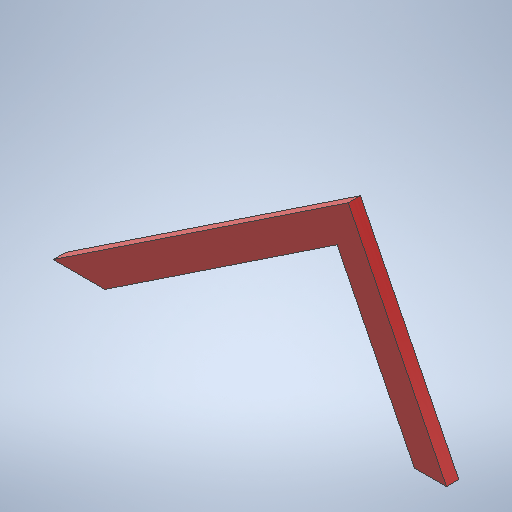
# Autodesk Inventor part: side1
Saved by Autodesk Inventor 2025.1 (Build 291241020, 241B)
## iProperties
Created: 2024-09-20
Part Number: side1
Material: Generic
Document SubType Name: Modeling
Designer: User
Density: 1 g/cm^3
Appearance: Default
Author: User
Autodesk Inventor part; units mm, degrees
ref_plane "YZ Plane" through (0, 0, 0) normal (1, 0, 0) x (0, 1, 0)
ref_plane "XZ Plane" through (0, 0, 0) normal (0, 1, 0) x (-1, 0, 0)
ref_plane "XY Plane" through (0, 0, 0) normal (0, 0, 1) x (1, 0, 0)
sketch "Sketch1" plane through (0, 0, 0) normal (0, 0, 1) x (1, 0, 0)
  line L0 (0, 0) -> (0, -38.1) projected
  line L1 (0, -38.1) -> (1219.2, -38.1) projected
  line L2 (1219.2, 0) -> (1219.2, -38.1) projected
  line L3 (0, 0) -> (1219.2, 0) projected
  line L4 (0, 0) -> (914.4, 0)
  line L5 (914.4, 609.6) -> (0, 0)
  line L6 (914.4, 609.6) -> (1219.2, 0)
  line L7 (1219.2, 0) -> (1126.19, 0)
  line L8 (1119.8068, 0) -> (879.9218, 479.77)
  line L9 (1119.8068, 0) -> (1219.2, 0)
  line L10 (160.2668, 0) -> (879.9218, 479.77)
  dimension "d3" = 88.9
  constraints: 14 end point, 4 point on line, 2 parallel, 1 collinear
  measures "d3" distance between parallel lines of L8 L6
extrude "Extrusion1" add sketch "Sketch1" against normal blind 38.1 contours L5 L6 L3 L8 L10
body "Solid1"
